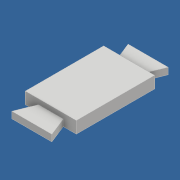
# Autodesk Inventor part: iPad_mount_center
Saved by Autodesk Inventor 2017 (Build 210142000, 142)
## iProperties
Part Number: iPad_mount_center
Material: 一般
Document SubType Name: Modeling
Designer: uhiit
Density: 1 g/cm^3
Appearance: 既定
Author: uhiit
Autodesk Inventor part; units mm, degrees
ref_plane "YZ Plane" through (0, 0, 0) normal (1, 0, 0) x (0, 1, 0)
ref_plane "XZ Plane" through (0, 0, 0) normal (0, 1, 0) x (-1, 0, 0)
ref_plane "XY Plane" through (0, 0, 0) normal (0, 0, 1) x (1, 0, 0)
sketch "スケッチ1" plane through (0, 0, 0) normal (0, 0, 1) x (1, 0, 0)
  line L0 (0, 10) -> (11.5, 10)
  line L1 (7.1451, -0.8872) -> (11.5, 10)
  line L2 (0, 10) -> (0, 0) construction
  line L3 (0, 10) -> (-11.5, 10)
  line L4 (-7.1451, -0.8872) -> (-11.5, 10)
  line L5 (7.1451, -0.8872) -> (7.1451, -45.8872)
  line L6 (-7.1451, -45.8872) -> (-7.1451, -0.8872)
  line L7 (-7.1451, -23.3872) -> (7.1451, -23.3872) construction
  line L8 (0, -56.7743) -> (11.5, -56.7743)
  line L9 (7.1451, -45.8872) -> (11.5, -56.7743)
  line L10 (0, -56.7743) -> (-11.5, -56.7743)
  line L11 (-7.1451, -45.8872) -> (-11.5, -56.7743)
  line L12 (7.1451, -0.8872) -> (7.1451, -45.8872)
  line L13 (7.1451, -45.8872) -> (11.5, -56.7743)
  line L14 (11.5, -56.7743) -> (-11.5, -56.7743)
  line L15 (-11.5, -56.7743) -> (-7.1451, -45.8872)
  line L16 (-7.1451, -45.8872) -> (-7.1451, -0.8872)
  line L17 (-7.1451, -0.8872) -> (-11.5, 10)
  line L18 (-11.5, 10) -> (11.5, 10)
  line L19 (11.5, 10) -> (7.1451, -0.8872)
  dimension "d0" = 7.2
  dimension "d1" = 11.5
  dimension "d3" = 45
  constraints: 40 end point, 6 symmetric about line, 4 equal length, 2 horizontal, 2 midpoint, 2 perpendicular, 2 vertical, 1 coincident
  measures "d0" distance of L2.end L1.start
  measures "d1" distance of L0.start L0.end
  measures "d3" distance of L5.start L5.end
extrude "押し出し1" add sketch "スケッチ1" along normal blind 3.8
sketch "スケッチ2" plane through (0, 0, 3.8) normal (0, 0, 1) x (1, 0, 0)
  line L0 (-11.5, 10) -> (-7.1451, -0.8872) projected
  line L1 (-7.1451, -0.8872) -> (-14.6451, -0.8872)
  line L2 (-14.6451, -0.8872) -> (-14.6451, -45.8872)
  line L3 (-14.6451, -45.8872) -> (-7.1451, -45.8872)
  line L4 (-7.1451, -45.8872) -> (-7.1451, -0.8872)
  line L5 (7.1451, -45.8872) -> (7.1451, -0.8872) projected
  line L6 (7.1451, -0.8872) -> (14.6451, -0.8872)
  line L7 (14.6451, -0.8872) -> (14.6451, -45.8872)
  line L8 (14.6451, -45.8872) -> (7.1451, -45.8872)
  line L9 (7.1451, -45.8872) -> (7.1451, -0.8872)
  point P0 (0, 0)
  dimension "d6" = 7.5
  dimension "d7" = 45
  dimension "d8" = 7.5
  constraints: 16 end point, 4 parallel, 2 horizontal, 2 perpendicular
  measures "d6" distance of L3.end L2.end
  measures "d7" distance of L2.end L1.end
  measures "d8" distance of L7.end L8.end
extrude "押し出し2" add sketch "スケッチ2" against normal blind 3.8
sketch "スケッチ3" plane through (0, 0, 3.8) normal (0, 0, 1) x (1, 0, 0)
  line L0 (14.6451, -0.8872) -> (14.6451, -45.8872) projected
  line L1 (-7.1451, -45.8872) -> (-14.6451, -45.8872) projected
  line L2 (14.6451, -0.8872) -> (-14.6451, -0.8872)
  line L3 (-14.6451, -0.8872) -> (-14.6451, -45.8872)
  line L4 (-14.6451, -45.8872) -> (14.6451, -45.8872)
  line L5 (14.6451, -45.8872) -> (14.6451, -0.8872)
  point P0 (0, 0)
  constraints: 8 end point, 2 parallel, 1 horizontal, 1 perpendicular
extrude "押し出し3" add sketch "スケッチ3" along normal blind 3
